Support motor rotor 2 (Autodesk Fusion 360 design; units mm, degrees)
Autodesk Fusion 360 part; units mm, degrees
note: some values were not read from the file. Chosen so that the rebuilt part matches the saved one: a direction. Set by a fixed rule: which sketch regions a step uses.
sketch "Sketch1" plane through (0, 0, 0) normal (0, 0, 1) x (1, 0, 0) in component "Component"
  circle A0 centre (0, 0) radius 12.5
  circle A1 centre (0, 0) radius 15
  circle A2 centre (0, 0) radius 16
  circle A3 centre (0, 0) radius 1.75
  dimension "d1" = 25
  dimension "d2" = 30
  dimension "d3" = 32
  dimension "d6" = 3.5
  constraint coincident A0.centre A1.centre
  constraint concentric A0 A1
  constraint concentric A0 A3
  measures "d1" diameter of A0
  measures "d2" diameter of A1
  measures "d3" diameter of A2
  measures "d6" diameter of A3
  measures "d16" diameter of A0.centre
extrude "Extrude1" add sketch "Sketch1" along normal blind 32 contours A1 makes body 1 in component "Component"
extrude "Extrude2" add sketch "Sketch1" against normal blind 2 contours A0 | A1 | A2 bodies 1 in component "Component"
sketch "Sketch2" plane through (0, 0, -2) normal (0, 0, -1) x (1, 0, 0) in component "Component"
  circle A0 centre (0, 0) radius 1.75
  circle A1 centre (0, 0) radius 16
  line L0 (1.6, -17.5) -> (-1.6, -17.5)
  line L1 (-1.6, -17.5) -> (-1.6, 17.5)
  line L2 (-1.6, 17.5) -> (1.6, 17.5)
  line L3 (1.6, 17.5) -> (1.6, -17.5)
  line L4 (1.6, -17.5) -> (-1.6, 17.5) construction
  line L5 (-1.6, -17.5) -> (1.6, 17.5) construction
  circle A2 centre (0, 0) radius 7.5
  dimension "d9" = 35
  dimension "d10" = 3.2
  dimension "d11" = 15
  constraint perpendicular L0 L1
  constraint parallel L0 L2
  constraint parallel L1 L3
  constraint horizontal L0
  constraint coincident L4 A0.centre
  constraint coincident L5 A0.centre
  constraint coincident A0.centre A1.centre
  measures "d9" distance of L0.end L1.end
  measures "d10" distance of L1.end L2.end
  measures "d11" diameter of A2
extrude "Extrude3" cut sketch "Sketch2" against normal blind 3 contours A1 L1 L3 A2 | A1 L1 L3 A2 bodies 1 in component "Component"
sketch "Sketch1 (2)" plane through (0, 0, 0) normal (0, 0, 1) x (1, 0, 0) in component "Component'"
  circle A0 centre (0, 0) radius 12.4
  circle A1 centre (0, 0) radius 18
  circle A2 centre (0, 0) radius 2.25
  dimension "d14" = 24.8
  dimension "d16" = 36
  dimension "d85" = 4.5
  constraint coincident A0.centre A1.centre
  constraint concentric A1 A2
  measures "d14" diameter of A0
  measures "d16" diameter of A1
  measures "d85" diameter of A2
extrude "Extrude1'" add sketch "Sketch1 (2)" along normal mid plane 6 separate body contours A1 makes body 2 in component "Component'"
extrude "Extrude2'" add sketch "Sketch1 (2)" along normal mid plane 16 contours A0 bodies 2 in component "Component'"
sketch "Sketch1 (3)" plane through (0, 0, 0) normal (0, 0, 1) x (1, 0, 0) in component "Component''"
  circle A0 centre (0, 0) radius 20
  circle A1 centre (0, 0) radius 12.5
  dimension "d21" = 40
  dimension "d22" = 25
  constraint coincident A0.centre A1.centre
  measures "d21" diameter of A0
  measures "d22" diameter of A1
extrude "Extrude1''" add sketch "Sketch1 (3)" along normal blind 5 separate body makes body 3 in component "Component''"
ref_plane "WorkPlane1" through (10, 0, 0) normal (1, 0, 0) x (0, 1, 0) in component "Component''"
sketch "Sketch2 (2)" plane through (10, 0, 0) normal (1, 0, 0) x (0, 1, 0) in component "Component''"
  line L0 (0, 0) -> (0, 65.3075) construction
  line L1 (20, 5) -> (-20, 5)
  line L2 (-15, 5) -> (-15, 23)
  line L3 (15, 5) -> (15, 23)
  arc A0 (15, 23) -> (-15, 23) centre (0, 23) ccw
  line L4 (12, 5) -> (12, 23)
  arc A1 (12, 23) -> (-12, 23) centre (0, 23) ccw
  line L5 (-12, 5) -> (-12, 23)
  circle A2 centre (0, 23) radius 3.5
  dimension "d26" = 30
  dimension "d27" = 18
  dimension "d28" = 3
  dimension "d35" = 7
  constraint coincident L0.start origin
  constraint vertical L0
  constraint coincident L0 A0.centre
  constraint coincident L1 L2.start
  constraint perpendicular L1 L2
  constraint coincident L1 L3.start
  constraint perpendicular L1 L3
  constraint tangent L3 A0
  constraint tangent L2 A0
  constraint concentric A0 A2
  measures "d26" diameter of A0
  measures "d27" distance of A0.centre L1
  measures "d35" diameter of A2
extrude "Extrude2''" add sketch "Sketch2 (2)" against normal blind 20 contours L1 L2 L3 A0 L4 A1 L5 bodies 3 in component "Component''"
sketch "Sketch3" plane through (0, -15, 0) normal (0, -1, 0) x (1, 0, 0) in component "Component''"
  line L0 (10, 5) -> (10, 23)
  line L1 (10, 23) -> (-10, 23)
  line L2 (-10, 23) -> (-10, 5)
  line L3 (-10, 5) -> (10, 5)
  line L4 (10, 23) -> (10, 38)
  line L5 (10, 38) -> (7, 38)
  line L6 (7, 38) -> (-10, 5)
  line L7 (-10, 5) -> (-10, 38)
  line L8 (-10, 38) -> (7, 38)
  dimension "d31" = 3
  constraint coincident L4.end L5.start
  constraint perpendicular L4 L5
  constraint coincident L2.end L3.start
  constraint perpendicular L1 L7
  constraint perpendicular L7 L8
  measures "d31" distance of L4.end L5.end
extrude "Extrude3'" cut sketch "Sketch3" against normal through all contours L1 L2 L6 L7 | L1 L6 L7 L8 bodies 3 in component "Component''"
extrude "Extrude4" add sketch "Sketch2 (2)" against normal blind 4.5 contours L1 L4 A1 L5 bodies 3 in component "Component''"
sketch "Sketch4" plane through (5.5, 0, 0) normal (-1, 0, 0) x (0, -1, 0) in component "Component''"
  circle A0 centre (0, 23) radius 3.5
  line L0 (-12, 23) -> (-12, 5)
  line L1 (-12, 5) -> (-11.225, 5)
  line L2 (-11.225, 5) -> (11.225, 5)
  line L3 (11.225, 5) -> (12, 5)
  line L4 (12, 5) -> (12, 23)
  arc A1 (12, 23) -> (-12, 23) centre (0, 23) ccw
  circle A2 centre (0, 23) radius 6.75
  dimension "d72" = 13.5
  constraint concentric A0 A2
  measures "d72" diameter of A2
extrude "Extrude5" cut sketch "Sketch4" against normal blind 3 contours A2 bodies 3 in component "Component''"
sketch "Sketch5" plane through (10, 0, 0) normal (1, 0, 0) x (0, 1, 0) in component "Component''"
  circle A0 centre (0, 23) radius 3.5
  line L0 (-15, 5) -> (-7.5, 5)
  line L1 (-7.5, 5) -> (7.5, 5)
  line L2 (7.5, 5) -> (15, 5)
  line L3 (15, 5) -> (15, 23)
  arc A1 (15, 23) -> (-15, 23) centre (0, 23) ccw
  line L4 (-15, 23) -> (-15, 5)
  line L5 (-15, 5) -> (15, 5)
  line L6 (15, 5) -> (15, 8)
  line L7 (15, 8) -> (-15, 8)
  line L8 (-15, 8) -> (-15, 5)
  circle A2 centre (0, 23) radius 8 construction
  line L9 (0, 23) -> (0, 38) construction
  circle A3 centre (0, 31) radius 1.25
  line L10 (0, 23) -> (-15, 23) construction
  circle A4 centre (-8, 23) radius 1.25
  line L11 (0, 23) -> (0, 8) construction
  circle A5 centre (0, 15) radius 1.25
  line L12 (0, 23) -> (15, 23) construction
  circle A6 centre (8, 23) radius 1.25
  dimension "d75" = 3
  dimension "d80" = 16
  dimension "d81" = 2.5
  dimension "d83" = 360
  constraint horizontal L5
  constraint vertical L6
  constraint horizontal L7
  constraint vertical L8
  constraint coincident L0.start L4.end
  constraint concentric A0 A2
  constraint coincident A0.centre A1.centre
  constraint midpoint A1 L9.end
  constraint coincident A2 A3.centre
  constraint coincident L9 A3.centre
  measures "d75" distance of L0.start L7.end
  measures "d80" diameter of A2
  measures "d81" diameter of A3
extrude "Extrude6" add sketch "Sketch5" along normal blind 3 contours L0 L1 L2 L3 L4 L5 L6 L7 L8 bodies 3 in component "Component''"
fillet "Fillet1" radius 32.5 1 edges at (13, 0, 8) on bodies 3 in component "Component''"
fillet "Fillet2" radius 3 1 edges at (10, 0, 8) on bodies 3 in component "Component''"
extrude "Extrude7" cut sketch "Sketch5" against normal through all contours A3 | A4 | A5 | A6 bodies 3 in component "Component''"
sketch "Sketch2 (3)" plane through (0, 0, 8) normal (0, 0, 1) x (-1, 0, 0) in component "Component'"
  circle A0 centre (0, 0) radius 2.25
  circle A1 centre (0, 0) radius 12.4
  circle A2 centre (0, 0) radius 7.5
  dimension "d86" = 15
  constraint coincident A0.centre A1.centre
  measures "d86" diameter of A2
extrude "Extrude3''" cut sketch "Sketch2 (3)" against normal blind 5 contours A2 bodies 2 in component "Component'"
component "Component" placed x (1, 0, 0) y (0, 1, 0) z (0, 0, 1) at (0, 0, 0)
component "Component'" placed x (1, 0, 0) y (0, 1, 0) z (0, 0, 1) at (0, 0, 35)
component "Component''" placed x (1, 0, 0) y (0, 1, 0) z (0, 0, 1) at (0, 0, 38)
